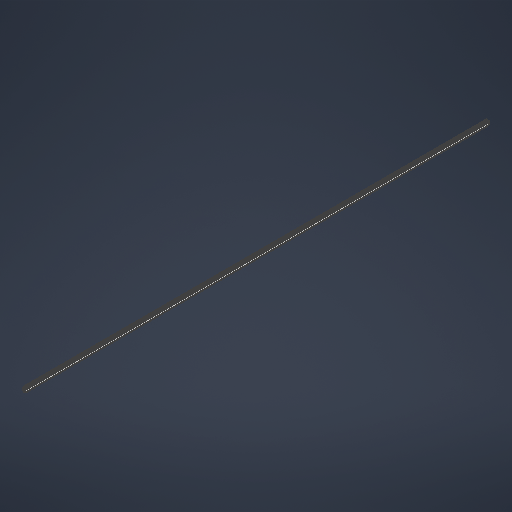
# Autodesk Inventor part: SP40-10 HOJA CORREDERA
Saved by Autodesk Inventor 2025 (Build 290162000, 162)
## iProperties
Created: 2026-01-18
Part Number: SP40-10 HOJA CORREDERA
Material: Aluminio
Document SubType Name: Modeling
Designer: ROLANDO
Density: 2.7 g/cm^3
Appearance: Satinado
Author: ROLANDO
Autodesk Inventor part; units mm, degrees
ref_plane "YZ Plane" through (0, 0, 0) normal (1, 0, 0) x (0, 1, 0)
ref_plane "XZ Plane" through (0, 0, 0) normal (0, 1, 0) x (-1, 0, 0)
ref_plane "XY Plane" through (0, 0, 0) normal (0, 0, 1) x (1, 0, 0)
sketch "Boceto1" plane through (0, 0, 0) normal (0, 0, 1) x (1, 0, 0)
  line L0 (28.1174, 40.2149) -> (1.9174, 40.2149)
  line L1 (1.9174, 41.6149) -> (28.1174, 41.6149)
  line L2 (0.0174, 0.0149) -> (0.0174, 51.8749)
  line L3 (24.8174, 56.0149) -> (24.8174, 54.3749)
  line L4 (28.6174, 54.6149) -> (28.6174, 48.1149)
  line L5 (28.6174, 46.7149) -> (24.8174, 46.7149)
  line L6 (24.8174, 46.7149) -> (24.8174, 48.3549)
  line L7 (26.2174, 48.1149) -> (28.6174, 48.1149)
  line L8 (26.2174, 49.3649) -> (25.5116, 49.3649)
  line L9 (25.5116, 49.3649) -> (24.8174, 48.3549)
  line L10 (26.2174, 53.3649) -> (25.5116, 53.3649)
  line L11 (1.4174, 42.1149) -> (1.4174, 49.1149)
  line L12 (1.4174, 49.1149) -> (2.9174, 49.1149)
  line L13 (2.9174, 49.1149) -> (2.9174, 51.8749)
  line L14 (4.1574, 56.0149) -> (10.8174, 56.0149)
  line L15 (9.3794, 54.6149) -> (5.6574, 54.6149)
  line L16 (10.8174, 56.0149) -> (10.8174, 53.5149)
  line L17 (10.8174, 53.5149) -> (10.1074, 53.5149)
  line L18 (10.1074, 53.5149) -> (9.3794, 54.6149)
  line L19 (26.2174, 54.6149) -> (28.6174, 54.6149)
  arc A0 (5.6574, 54.6149) -> (2.9174, 51.8749) centre (5.6574, 51.8749) ccw
  arc A1 (4.1574, 56.0149) -> (0.0174, 51.8749) centre (4.1574, 51.8749) ccw
  line L20 (24.8174, 54.3749) -> (25.5116, 53.3649)
  line L21 (26.2174, 54.6149) -> (26.2174, 53.3649)
  line L22 (26.2174, 48.1149) -> (26.2174, 49.3649)
  arc A2 (1.9174, 40.2149) -> (1.4174, 39.7149) centre (1.9174, 39.7149) ccw
  arc A3 (28.6174, 39.7149) -> (28.1174, 40.2149) centre (28.1174, 39.7149) ccw
  arc A4 (28.1174, 41.6149) -> (28.6174, 42.1149) centre (28.1174, 42.1149) ccw
  arc A5 (1.4174, 42.1149) -> (1.9174, 41.6149) centre (1.9174, 42.1149) ccw
  line L23 (30.0174, 56.0149) -> (24.8174, 56.0149)
  line L24 (28.6174, 42.1149) -> (28.6174, 46.7149)
  line L25 (30.0174, 56.0149) -> (30.0174, 0.0149)
  line L26 (1.4174, 29.2149) -> (28.6174, 29.2149)
  line L27 (1.4174, 27.8149) -> (28.6174, 27.8149)
  line L28 (1.4174, 39.7149) -> (1.4174, 29.2149)
  line L29 (1.4174, 27.8149) -> (1.4174, 1.4149)
  line L30 (28.6174, 1.4149) -> (28.6174, 27.8149)
  line L31 (28.6174, 29.2149) -> (28.6174, 39.7149)
  line L32 (28.6174, 39.7149) -> (28.6174, 29.2149)
  line L33 (28.6174, 27.8149) -> (28.6174, 1.4149)
  line L34 (4.5174, 6.1149) -> (6.8174, 6.1149)
  line L35 (7.8174, 5.1149) -> (7.8174, 2.7149)
  line L36 (7.8174, 2.7149) -> (6.4174, 2.7149)
  line L37 (6.4174, 2.7149) -> (6.4174, 4.7149)
  line L38 (6.4174, 4.7149) -> (4.9174, 4.7149)
  line L39 (4.9174, 4.7149) -> (4.9174, -3.2851)
  line L40 (4.9174, -3.2851) -> (6.4174, -3.2851)
  line L41 (6.4174, -3.2851) -> (6.4174, -1.2851)
  line L42 (6.4174, -1.2851) -> (7.8174, -1.2851)
  line L43 (7.8174, -1.2851) -> (7.8174, -3.6851)
  line L44 (6.8174, -4.6851) -> (3.5174, -4.6851)
  line L45 (3.5174, -4.6851) -> (3.5174, 0.0149)
  arc A6 (7.8174, 5.1149) -> (6.8174, 6.1149) centre (6.8174, 5.1149) ccw
  arc A7 (4.5174, 6.1149) -> (3.5174, 5.1149) centre (4.5174, 5.1149) ccw
  arc A8 (6.8174, -4.6851) -> (7.8174, -3.6851) centre (6.8174, -3.6851) ccw
  line L46 (3.5174, 1.4149) -> (1.4174, 1.4149)
  line L47 (3.5174, 0.0149) -> (0.0174, 0.0149)
  line L48 (3.5174, 1.4149) -> (3.5174, 5.1149)
  line L49 (25.5174, 6.1149) -> (23.2174, 6.1149)
  line L50 (22.2174, 5.1149) -> (22.2174, 2.7149)
  line L51 (22.2174, 2.7149) -> (23.6174, 2.7149)
  line L52 (23.6174, 2.7149) -> (23.6174, 4.7149)
  line L53 (23.6174, 4.7149) -> (25.1174, 4.7149)
  line L54 (25.1174, 4.7149) -> (25.1174, -3.2851)
  line L55 (25.1174, -3.2851) -> (23.6174, -3.2851)
  line L56 (23.6174, -3.2851) -> (23.6174, -1.2851)
  line L57 (23.6174, -1.2851) -> (22.2174, -1.2851)
  line L58 (22.2174, -1.2851) -> (22.2174, -3.6851)
  line L59 (23.2174, -4.6851) -> (26.5174, -4.6851)
  line L60 (26.5174, -4.6851) -> (26.5174, 0.0149)
  arc A9 (23.2174, 6.1149) -> (22.2174, 5.1149) centre (23.2174, 5.1149) ccw
  arc A10 (26.5174, 5.1149) -> (25.5174, 6.1149) centre (25.5174, 5.1149) ccw
  arc A11 (22.2174, -3.6851) -> (23.2174, -4.6851) centre (23.2174, -3.6851) ccw
  line L61 (26.5174, 1.4149) -> (28.6174, 1.4149)
  line L62 (26.5174, 0.0149) -> (30.0174, 0.0149)
  line L63 (26.5174, 1.4149) -> (26.5174, 5.1149)
  point P0 (28.6174, 51.3649)
  point P1 (0.0174, 0.9149)
  point P2 (4.9174, 0.7149)
  point P3 (25.1174, 0.7149)
  dimension "d31" = 1.4
  dimension "d42" = 2.5
  dimension "d43" = 0.71
  dimension "d45" = 2.9
  dimension "d47" = 33.5
  dimension "d48" = 7.5
  dimension "d51" = 2.74
  dimension "d59" = 6.9
  dimension "d60" = 1.4
  dimension "d78" = 6.5
  dimension "d84" = 1.4
  dimension "d85" = 1.4
  dimension "d88" = 2.4
  dimension "d95" = 6.02
  dimension "d99" = 111
  dimension "d100" = 2.4
  dimension "d109" = 0.7058
  dimension "d110" = 0.7058
  dimension "d143" = 1.4
  dimension "d147" = 1.4
  dimension "d148" = 30
  dimension "d149" = 1.4
  dimension "d150" = 14
  dimension "d151" = 27.2
  dimension "d152" = 14.4
  dimension "d153" = 1.4
  dimension "d154" = 11
  dimension "d155" = 1.4
  dimension "d156" = 1.4
  dimension "d157" = 1.4
  dimension "d158" = 1.4
  dimension "d162" = 60.7
  dimension "d163" = 10.8
  dimension "d164" = 8
  dimension "d165" = 2
  dimension "d166" = 4
  dimension "d167" = 1.5
  dimension "d168" = 7.8
  dimension "d169" = 1
  dimension "d172" = 1.4
  dimension "d173" = 4.7
  dimension "d175" = 56
  dimension "d176" = 13.8
  dimension "d177" = 14.4
  dimension "d180" = 1.5
  dimension "d181" = 4.14
  dimension "d182" = 10.8
  dimension "d183" = 14.4
  dimension "d184" = 0.5
  dimension "d187" = 3.5
  dimension "d188" = 4.9
  dimension "d189" = 6.4
  dimension "d190" = 7.8
  dimension "d191" = 26.5
  dimension "d193" = 54.6
  dimension "d195" = 3.5
  dimension "d196" = 4.9
  dimension "d197" = 53.9
  dimension "d198" = 53.7
  dimension "d199" = 2
  dimension "d200" = 2
  dimension "d201" = 4
  dimension "d202" = 3.01
  dimension "d203" = 9.3
  constraints: 128 end point, 29 tangent, 24 point on circle, 21 perpendicular, 13 parallel, 12 centre point, 12 collinear, 8 equal radius, 7 horizontal, 4 point on line, 4 vertical, 2 equal length, 2 midpoint
  measures "d31" distance between parallel lines of L15 L14
  measures "d42" distance of L14.end L16.end
  measures "d43" distance of L16.end L17.end
  measures "d45" distance between parallel lines of L13 L2
  measures "d47" angle of L16 L18
  measures "d48" distance between parallel lines of L1 L12
  measures "d51" radius of A0
  measures "d59" distance between parallel lines of L12 L14
  measures "d60" distance between parallel lines of L2 L11
  measures "d78" distance between parallel lines of L7 L19
  measures "d84" distance between parallel lines of L6 L22
  measures "d85" distance between parallel lines of L3 L21
  measures "d88" distance between parallel lines of L4 L21
  measures "d95" distance of L6.end L3.end
  measures "d99" angle of L9 L20
  measures "d100" distance between parallel lines of L4 L22
  measures "d109" distance of L10.start L10.end
  measures "d110" distance of L8.start L8.end
  measures "d143" distance between parallel lines of L1 L0
  measures "d147" distance between parallel lines of L7 L5
  measures "d148" distance between parallel lines of L25 L2
  measures "d149" distance between parallel lines of L25 L24
  measures "d150" distance between parallel lines of L3 L16
  measures "d151" distance between parallel lines of L4 L11
  measures "d152" distance between parallel lines of L1 L14
  measures "d153" distance between parallel lines of L27 L26
  measures "d154" distance between parallel lines of L26 L0
  measures "d155" distance between parallel lines of L35 L37
  measures "d156" distance between parallel lines of L34 L38
  measures "d157" distance between parallel lines of L43 L41
  measures "d158" distance between parallel lines of L44 L40
  measures "d162" distance between parallel lines of L44 L14
  measures "d163" distance between parallel lines of L44 L34
  measures "d164" distance between parallel lines of L40 L38
  measures "d165" distance from line of L36 point (4.917, 0.715)
  measures "d166" distance between parallel lines of L42 L36
  measures "d167" distance between parallel lines of L39 L37
  measures "d168" distance between parallel lines of L2 L43
  measures "d169" radius of A6
  measures "d172" distance between parallel lines of L46 L47
  measures "d173" distance between parallel lines of L34 L46
  measures "d175" distance between parallel lines of L14 L47
  measures "d176" distance between parallel lines of L27 L1
  measures "d177" distance between parallel lines of L23 L1
  measures "d180" distance of A0.centre A1.centre
  measures "d181" radius of A1
  measures "d182" distance between parallel lines of L16 L2
  measures "d183" distance between parallel lines of L58 L43
  measures "d184" radius of A4
  measures "d187" distance between parallel lines of L63 L25
  measures "d188" distance between parallel lines of L54 L25
  measures "d189" distance between parallel lines of L52 L25
  measures "d190" distance between parallel lines of L50 L25
  measures "d191" distance between parallel lines of L45 L25
  measures "d193" distance between parallel lines of L19 L62
  measures "d195" distance from line of L23.start L60
  measures "d196" distance from line of point (25.117, 0.715) L25
  measures "d197" distance from line of point (25.117, 0.715) L19
  measures "d198" distance from line of point (0.017, 0.915) L19
  measures "d199" distance from line of L10 point (28.617, 51.365)
  measures "d200" distance from line of point (28.617, 51.365) L8
  measures "d201" distance between parallel lines of L8 L10
  measures "d202" vertical distance of point (28.617, 51.365) L3.end
  measures "d203" distance between parallel lines of L5 L23
extrude "Extrusión1" add sketch "Boceto1" against normal blind 5800
